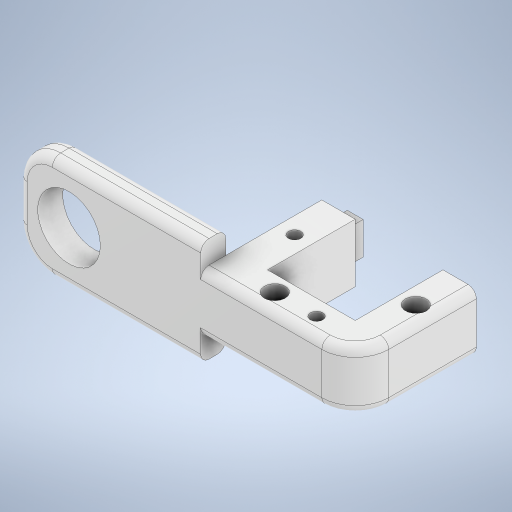
# Autodesk Inventor part: ServoMount
Saved by Autodesk Inventor 2024 (Build 280153000, 153)
## iProperties
Created: 2025-12-19
Part Number: ServoMount
Material: Generic
Document SubType Name: Modeling
Designer: Liam
Density: 1 g/cm^3
Appearance: Default
Mass: 16.9428 g
Surface Area: 79.0033 cm^2
Volume: 16.9428 cm^3
Author: Liam
Autodesk Inventor part; units mm, degrees
ref_plane "YZ Plane" through (0, 0, 0) normal (1, 0, 0) x (0, 1, 0)
sketch "Sketch1" plane through (0, 0, 0) normal (0, 1, 0) x (-1, 0, 0)
  line L0 (0, 0) -> (21, 0)
  circle A0 centre (5.5, 3.75) radius 1.5
  line L1 (29, 8) -> (-8, 8)
  line L2 (10.5, 8) -> (10.5, 0) construction
  line L3 (0, -21) -> (-8, -21)
  line L4 (29, 2) -> (72.5, 2)
  line L5 (72.5, 2) -> (72.5, 8)
  line L6 (72.5, 8) -> (29, 8)
  line L7 (29, 8) -> (29, 2)
  line L8 (21, 0) -> (21, 8)
  line L9 (0, 0) -> (0, 8)
  circle A1 centre (15.5, 3.75) radius 2.5
  line L10 (0, 0) -> (0, -21)
  line L11 (-8, -21) -> (-8, 8)
  line L12 (21, -21) -> (21, 0)
  line L13 (29, -21) -> (29, 2)
  line L14 (21, -21) -> (29, -21)
  circle A2 centre (-4, -10.5) radius 2.5
  circle A3 centre (25, -10.5) radius 1.5
  point P0 (29, 8)
  point P1 (21, 8)
  point P2 (-4, -21)
  dimension "d1" = 21
  dimension "d15" = 3.75
  dimension "d16" = 5
  dimension "d51" = 6
  dimension "d148" = 5
  dimension "d149" = 3.75
  dimension "d150" = 5
  dimension "d151" = 3
  dimension "d152" = 8
  dimension "d154" = 37
  dimension "d155" = 10.5
  dimension "d158" = 21
  dimension "d160" = 8
  dimension "d162" = 8
  dimension "d164" = 21
  dimension "d165" = 29
  dimension "d166" = 29
  dimension "d169" = 62
  dimension "d170" = 4
  dimension "d171" = 5
  dimension "d172" = 10.5
  dimension "d173" = 4
  dimension "d174" = 3
  dimension "d175" = 10.5
  constraints: 30 end point, 4 centre point, 4 parallel, 4 perpendicular, 3 horizontal, 3 midpoint, 1 vertical
  measures "d1" distance of L0.start L0.end
  measures "d15" distance from line of L0 A0.centre
  measures "d16" distance from line of L2 A0.centre
  measures "d51" distance of L4.end L5.end
  measures "d148" diameter of A1
  measures "d149" distance from line of L0 A1.centre
  measures "d150" distance from line of L2 A1.centre
  measures "d151" diameter of A0
  measures "d152" distance of L3.start L3.end
  measures "d154" distance between parallel lines of L13 L11
  measures "d155" distance between parallel lines of L9 L2
  measures "d158" distance from line of L0.start L3
  measures "d160" distance between parallel lines of L1 L0
  measures "d162" distance of L12.start L13.start
  measures "d164" distance between parallel lines of L0 L14
  measures "d165" distance of L3.end L1.end
  measures "d166" distance between parallel lines of L6 L14
  measures "d169" distance between parallel lines of L5 L2
  measures "d170" distance from line of L10 A2.centre
  measures "d171" diameter of A2
  measures "d172" distance of point (-4, -21) A2.centre
  measures "d173" distance from line of L12 A3.centre
  measures "d174" diameter of A3
  measures "d175" distance from line of L14 A3.centre
extrude "Extrusion1" add sketch "Sketch1" along normal mid plane 14 contours L9 L1 L8 L0 | L10 L3 L11 L1 L9 | L8 L1 L7 L13 L14 L12
extrude "Extrusion2" add sketch "Sketch1" along normal mid plane 25 contours L6 L5 L4 L7
fillet "Fillet4" radius 8 3 edges at (-72.5, 12.5, 5) (-72.5, -12.5, 5) (8, 0, 8)
ref_plane "Work Plane3" through (0, 0, 2) normal (0, 0, 1) x (1, 0, 0)
sketch "Sketch5" plane through (0, 0, 2) normal (0, 0, 1) x (1, 0, 0)
  line L0 (-29, -7) -> (-29, 7) projected
  circle A0 centre (-60.5, 0) radius 7.5
  line L1 (-21, -7) -> (0, -7) projected
  line L2 (-29, 12.5) -> (-64.5, 12.5) projected
  point P0 (0, 0)
  point P1 (-12.116, -8.0773)
  point P2 (-29, 0)
  point P3 (-10.5, -7)
  dimension "d195" = 15
  dimension "d196" = 50
  dimension "d197" = 12.5
  constraints: 2 midpoint, 1 centre point
  measures "d195" diameter of A0
  measures "d196" horizontal distance of point (-10.5, -7) A0.centre
  measures "d197" distance from line of L2 A0.centre
extrude "Extrusion6" cut sketch "Sketch5" along normal blind 6
fillet "Fillet12" radius 2 13 edges at (-72.5, 0, 8) (-46.75, 12.5, 8) (-70.1569, -10.1569, 2) (-72.5, 0, 2) (-70.1569, 10.1569, 2) (-46.75, 12.5, 2) (-46.75, -12.5, 2) (5.6569, 7, 5.6569) (8, 7, -10.5) (-14.5, 7, 8) (5.6569, -7, 5.6569) (8, -7, -10.5) (-14.5, -7, 8)
ref_plane "Work Plane4" through (0, 0, -21) normal (0, 0, 1) x (1, 0, 0)
sketch "Sketch6" plane through (0, 0, -21) normal (0, 0, 1) x (1, 0, 0)
  line L0 (6, -4) -> (2, -4)
  line L1 (2, -4) -> (2, 4)
  line L2 (2, 4) -> (6, 4)
  line L3 (6, 4) -> (6, -4)
  line L4 (6, -4) -> (2, 4) construction
  line L5 (2, -4) -> (6, 4) construction
  line L6 (0, -7) -> (0, 7) projected
  line L7 (-23.1, -3.9) -> (-26.9, -3.9)
  line L8 (-26.9, -3.9) -> (-26.9, 3.9)
  line L9 (-26.9, 3.9) -> (-23.1, 3.9)
  line L10 (-23.1, 3.9) -> (-23.1, -3.9)
  line L11 (-23.1, -3.9) -> (-26.9, 3.9) construction
  line L12 (-26.9, -3.9) -> (-23.1, 3.9) construction
  line L13 (-21, -7) -> (-21, 7) projected
  point P0 (0, 0)
  point P1 (4, 0)
  point P2 (0, 0)
  point P3 (0, 0)
  point P4 (-25, 0)
  point P5 (-21, 0)
  dimension "d183" = 8
  dimension "d184" = 4
  dimension "d185" = 4
  dimension "d186" = 0
  dimension "d187" = 7.8
  dimension "d188" = 3.8
  dimension "d189" = 4
  dimension "d190" = 0
  constraints: 24 end point, 7 midpoint, 4 parallel, 2 horizontal, 2 perpendicular
  measures "d183" distance of L2.end L0.start
  measures "d184" distance of L1.end L2.end
  measures "d185" distance of point (4, 0) point (0, 0)
  measures "d186" vertical distance of point (0, 0) point (4, 0)
  measures "d187" distance of L7.end L8.end
  measures "d188" distance of L8.end L9.end
  measures "d189" distance from line of L13 point (-25, 0)
  measures "d190" vertical distance of point (-21, 0) point (-25, 0)
extrude "Extrusion12" add sketch "Sketch6" against normal blind 4 contours L7 L8 L9 L10
extrude "Extrusion13" cut sketch "Sketch6" along normal blind 4 contours L0 L1 L2 L3
equation "\"HoleDiameter\" = 3"
equation "\"InsertDiameter\" = 5"
equation "\"CoxaWidth\" = 25"
equation "\"SlotWidth1\" = 4"
equation "\"SlotLength1\" = 8"
equation "\"SlotHeight1\" = 4"
body "Solid1"
